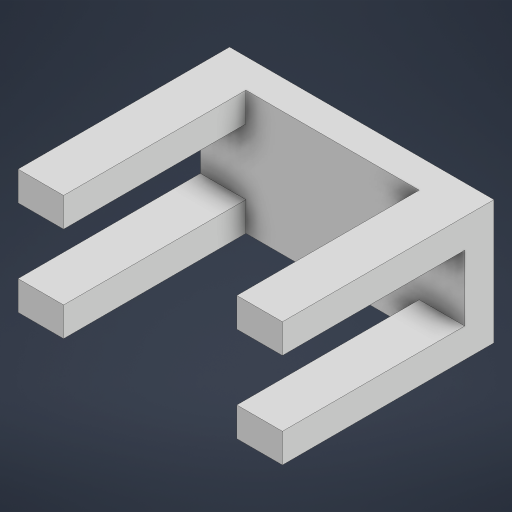
# Autodesk Inventor part: ButtonLock
Saved by Autodesk Inventor 2024.2 (Build 282272000, 272)
## iProperties
Created: 2024-06-06
Part Number: ButtonLock
Material: Generic
Document SubType Name: Modeling
Designer: simon
Density: 1 g/cm^3
Appearance: Default
Author: simon
Autodesk Inventor part; units mm, degrees
ref_plane "YZ Plane" through (0, 0, 0) normal (1, 0, 0) x (0, 1, 0)
ref_plane "XZ Plane" through (0, 0, 0) normal (0, 1, 0) x (-1, 0, 0)
ref_plane "XY Plane" through (0, 0, 0) normal (0, 0, 1) x (1, 0, 0)
sketch "Sketch1" plane through (0, 0, 0) normal (0, 0, 1) x (1, 0, 0)
  line L0 (0, 0) -> (14.5, 0)
  line L1 (14.5, 0) -> (14.5, 6.8)
  line L2 (14.5, 6.8) -> (0, 6.8)
  line L3 (0, 6.8) -> (0, 0)
  dimension "d0" = 14.5
  dimension "d1" = 6.8
  constraints: 8 end point, 2 parallel, 1 horizontal, 1 perpendicular
  measures "d0" distance of L2.end L1.end
  measures "d1" distance of L1.end L0.end
extrude "Extrusion1" add sketch "Sketch1" along normal blind 1.6
sketch "Sketch2" plane through (0, 0, 1.6) normal (0, 0, 1) x (1, 0, 0)
  line L0 (0, 6.8) -> (0, 0) projected
  line L1 (0, 6.8) -> (2.5, 6.8)
  line L2 (2.5, 6.8) -> (2.5, 5.2)
  line L3 (2.5, 5.2) -> (0, 5.2)
  line L4 (0, 5.2) -> (0, 6.8)
  line L5 (0, 0) -> (2.5, 0)
  line L6 (2.5, 0) -> (2.5, 1.6)
  line L7 (2.5, 1.6) -> (0, 1.6)
  line L8 (0, 1.6) -> (0, 0)
  line L9 (0, 0) -> (14.5, 0) projected
  line L10 (14.5, 0) -> (12, 0)
  line L11 (12, 0) -> (12, 1.6)
  line L12 (12, 1.6) -> (14.5, 1.6)
  line L13 (14.5, 1.6) -> (14.5, 0)
  line L14 (14.5, 0) -> (14.5, 6.8) projected
  line L15 (14.5, 6.8) -> (12, 6.8)
  line L16 (12, 6.8) -> (12, 5.2)
  line L17 (12, 5.2) -> (14.5, 5.2)
  line L18 (14.5, 5.2) -> (14.5, 6.8)
  dimension "d4" = 2.5
  dimension "d5" = 1.6
  dimension "d6" = 2.5
  dimension "d7" = 1.6
  dimension "d8" = 2.5
  dimension "d9" = 1.6
  dimension "d10" = 1.6
  constraints: 32 end point, 8 parallel, 4 horizontal, 4 perpendicular, 1 point on line
  measures "d4" distance of L2.end L3.end
  measures "d5" distance of L1.end L2.end
  measures "d6" distance of L7.end L6.end
  measures "d7" distance of L6.end L5.end
  measures "d8" distance of L11.end L12.end
  measures "d9" distance of L10.end L11.end
  measures "d10" distance of L16.end L15.end
extrude "Extrusion2" add sketch "Sketch2" along normal blind 10
body "Solid1"
